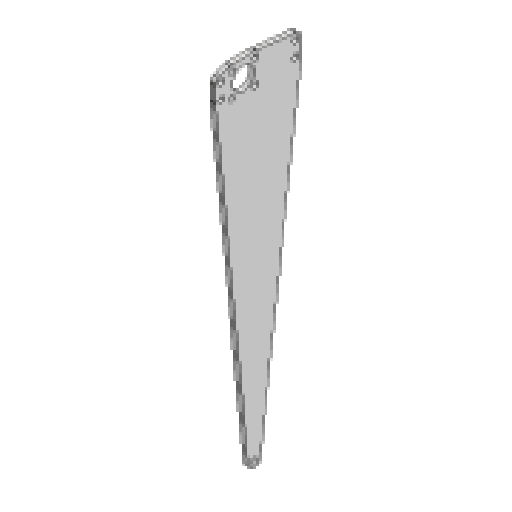
# Autodesk Inventor part: IntakeSlidePlate1.0
Saved by Autodesk Inventor 2023 (Build 270158000, 158)
## iProperties
Created: 2022-10-12
Part Number: IntakeSlidePlate1.0
Material: Generic
Document SubType Name: Modeling
Designer: deli
Density: 1 g/cm^3
Appearance: Default
Author: deli
Autodesk Inventor part; units mm, degrees
ref_plane "YZ Plane" through (0, 0, 0) normal (1, 0, 0) x (0, 1, 0)
ref_plane "XZ Plane" through (0, 0, 0) normal (0, 1, 0) x (-1, 0, 0)
ref_plane "XY Plane" through (0, 0, 0) normal (0, 0, 1) x (1, 0, 0)
sketch "Sketch1" plane through (0, 0, 0) normal (1, 0, 0) x (0, 1, 0)
  circle A0 centre (-139.9183, -37.2831) radius 2
  arc A1 (-140.7097, -33.3622) -> (-140.9001, -41.1608) centre (-139.9183, -37.2831) ccw
  line L0 (-31.7097, -11.3622) -> (-140.7097, -33.3622)
  line L1 (-31.9001, -68.7608) -> (-140.9001, -41.1608)
  line L2 (-30.9183, -11.2831) -> (-20.9183, -11.2831)
  line L3 (-30.9183, -68.8831) -> (-20.9183, -68.8831)
  circle A2 centre (-25.9183, -30.0831) radius 7.5
  circle A3 centre (-30.9183, -15.2831) radius 2
  circle A4 centre (-20.9183, -15.2831) radius 2
  arc A5 (-17.2586, -13.6686) -> (-20.9183, -11.2831) centre (-20.9183, -15.2831) ccw
  circle A6 centre (-20.9183, -64.8831) radius 2
  circle A7 centre (-30.9183, -64.8831) radius 2
  arc A8 (-31.9001, -68.7608) -> (-30.9183, -68.8831) centre (-30.9183, -64.8831) ccw
  arc A9 (-20.9183, -68.8831) -> (-16.9431, -65.3281) centre (-20.9183, -64.8831) ccw
  arc A10 (-30.9183, -11.2831) -> (-31.7097, -11.3622) centre (-30.9183, -15.2831) ccw
  line L4 (-50.4183, -15.1382) -> (-50.4183, -64.0718) construction
  line L5 (-59.4183, -16.9548) -> (-59.4183, -61.7929) construction
  circle A11 centre (-17.9183, -22.0831) radius 2
  circle A12 centre (-17.9183, -38.0831) radius 2
  circle A13 centre (-33.9183, -22.0831) radius 2
  circle A14 centre (-33.9183, -38.0831) radius 2
  line L6 (-17.9183, -22.0831) -> (-17.9183, -38.0831) construction
  line L7 (-17.9183, -38.0831) -> (-33.9183, -38.0831) construction
  line L8 (-33.9183, -38.0831) -> (-33.9183, -22.0831) construction
  line L9 (-33.9183, -22.0831) -> (-17.9183, -22.0831) construction
  circle A15 centre (-25.9183, -30.0831) radius 9.3137 construction
  line L10 (-13.9183, -22.0831) -> (-13.9183, -38.0831)
  line L11 (-14.2586, -20.4686) -> (-17.2586, -13.6686)
  arc A16 (-13.9183, -22.0831) -> (-14.2586, -20.4686) centre (-17.9183, -22.0831) ccw
  line L12 (-13.9431, -38.5281) -> (-16.9431, -65.3281)
  arc A17 (-13.9431, -38.5281) -> (-13.9183, -38.0831) centre (-17.9183, -38.0831) ccw
  point P0 (0, 0)
  dimension "d2" = 4
  dimension "d5" = 8
  dimension "d11" = 26
  dimension "d12" = 15
  dimension "d14" = 4
  dimension "d15" = 14.8
  dimension "d16" = 10
  dimension "d17" = 4
  dimension "d18" = 5
  dimension "d19" = 10
  dimension "d20" = 49.6
  dimension "d21" = 49.6
  dimension "d23" = 9
  dimension "d25" = 80.5
  dimension "d29" = 16
  dimension "d31" = 0
  dimension "d32" = 19.5
  dimension "d33" = 36.5
  constraints: 26 end point, 18 centre point, 16 tangent, 14 point on circle, 12 equal radius, 8 coincident, 4 perpendicular, 4 point on line, 3 horizontal, 1 parallel, 1 vertical
  measures "d2" diameter of A0
  measures "d5" diameter of A1
  measures "d11" distance from line of A0.centre L2
  measures "d12" diameter of A2
  measures "d14" distance from line of L2 A3.centre
  measures "d15" vertical distance of A2.centre A3.centre
  measures "d16" distance of A3.centre A4.centre
  measures "d17" distance from line of L2 A4.centre
  measures "d18" horizontal distance of A2.centre A3.centre
  measures "d19" distance of A7.centre A6.centre
  measures "d20" distance of A6.centre A4.centre
  measures "d21" distance of A7.centre A3.centre
  measures "d23" distance between parallel lines of L4 L5
  measures "d25" distance from line of A0.centre L5
  measures "d29" distance of L6.start L6.end
  measures "d31" horizontal distance of A6.centre A4.centre
  measures "d32" distance from line of A3.centre L4
  measures "d33" distance between parallel lines of L4 L10
extrude "Extrusion1" add sketch "Sketch1" along normal blind 3.175
equation "\"d17\" = d14"
equation "\"d18\" = 0.5 * d16"
equation "\"d19\" = d16"
equation "\"d21\" = d20"
body "Solid1"
